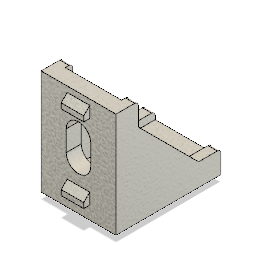
2020 Corner Bracket v1 (Autodesk Fusion 360 design; units mm, degrees)
Autodesk Fusion 360 part; units mm, degrees
sketch "Sketch1" plane through (0, 0, 0) normal (1, 0, 0) x (0, 0, -1)
  line L0 (0, 0) -> (0, 28)
  line L1 (0, 28) -> (5, 28)
  line L2 (6, 27) -> (6, 22)
  line L3 (6, 22) -> (22, 6)
  line L4 (22, 6) -> (27, 6)
  line L5 (28, 5) -> (28, 0)
  line L6 (28, 0) -> (0, 0)
  line L7 (4, 4) -> (28, 4)
  line L8 (4, 4) -> (4, 28)
  arc A0 (6, 27) -> (5, 28) centre (5, 27) ccw
  arc A1 (28, 5) -> (27, 6) centre (27, 5) ccw
  line L9 (0, 26.5) -> (-1.6, 24.9)
  line L10 (-1.6, 24.9) -> (-1.6, 23.5)
  line L11 (-1.6, 23.5) -> (0, 23.5)
  line L12 (0, 6.5) -> (-1.6, 4.9)
  line L13 (-1.6, 4.9) -> (-1.6, 3.5)
  line L14 (-1.6, 3.5) -> (0, 3.5)
  line L15 (3.5, 0) -> (3.5, -1.6)
  line L16 (3.5, -1.6) -> (4.9, -1.6)
  line L17 (4.9, -1.6) -> (6.5, 0)
  line L18 (23.5, 0) -> (23.5, -1.6)
  line L19 (23.5, -1.6) -> (24.9, -1.6)
  line L20 (24.9, -1.6) -> (26.5, 0)
  line L21 (-56.6063, 27.9695) -> (-36.6063, 27.9695)
  line L22 (-36.6063, 27.9695) -> (-36.6063, -0.0305)
  line L23 (-36.6063, -0.0305) -> (-56.6063, -0.0305)
  line L24 (-56.6063, -0.0305) -> (-56.6063, 27.9695)
  line L25 (-54.1063, 3.9695) -> (-39.1063, 3.9695)
  line L26 (-39.1063, 3.9695) -> (-39.1063, 27.9695)
  line L27 (-39.1063, 27.9695) -> (-54.1063, 27.9695)
  line L28 (-54.1063, 27.9695) -> (-54.1063, 3.9695)
  line L29 (-49.7743, 13.4695) -> (-49.7743, 16.9695)
  arc A2 (-43.2743, 16.9695) -> (-49.7743, 16.9695) centre (-46.5243, 16.9695) ccw
  line L30 (-43.2743, 16.9695) -> (-43.2743, 13.4695)
  arc A3 (-49.7743, 13.4695) -> (-43.2743, 13.4695) centre (-46.5243, 13.4695) ccw
  line L31 (-49.5243, -1.6305) -> (-43.5243, -1.6305)
  line L32 (-43.5243, -1.6305) -> (-43.5243, -0.0305)
  line L33 (-43.5243, -0.0305) -> (-49.5243, -0.0305)
  line L34 (-49.5243, -0.0305) -> (-49.5243, -1.6305)
  point P0 (6, 28)
  point P1 (28, 6)
  dimension "d1" = 28
  dimension "d2" = 28
  dimension "d3" = 6
  dimension "d4" = 6
  dimension "d5" = 45
  dimension "d6" = 22
  dimension "d7" = 4
  dimension "d8" = 4
  dimension "d9" = 1
  dimension "d11" = 45
  dimension "d12" = 1.6
  dimension "d14" = 3
  dimension "d16" = 3
  dimension "d17" = 20
  dimension "d18" = 20
  dimension "d19" = 3
  dimension "d20" = 3
  dimension "d21" = 45
  dimension "d22" = 3.5
  dimension "d23" = 1.6
  dimension "d26" = 20
  dimension "d27" = 2.5
  dimension "d28" = 15
  dimension "d29" = 6.5
  dimension "d30" = 3.5
  dimension "d31" = 13.5
  dimension "d32" = 4
  dimension "d33" = 28
  dimension "d34" = 6
  dimension "d35" = 0.25
  dimension "d36" = 1.6
  dimension "d41" = 3.5
  constraint coincident L0.start L6.end
  constraint vertical L0
  constraint perpendicular L0 L1
  constraint perpendicular L1 L2
  constraint perpendicular L2 L4
  constraint perpendicular L4 L5
  constraint perpendicular L0 L6
  constraint coincident L5 L7.end
  constraint perpendicular L5 L7
  constraint coincident L1 L8.end
  constraint perpendicular L1 L8
  constraint coincident P0 L1
  constraint coincident P0 L2
  constraint tangent L1 A0
  constraint tangent L2 A0
  constraint coincident P1 L4
  constraint coincident P1 L5
  constraint tangent L4 A1
  constraint tangent L5 A1
  constraint equal A0 A1
  constraint coincident L0 L9.start
  constraint parallel L0 L10
  constraint coincident L0 L11.end
  constraint perpendicular L0 L11
  constraint coincident L0 L12.start
  constraint parallel L0 L13
  constraint coincident L0 L14.end
  constraint perpendicular L0 L14
  constraint collinear L10 L13
  constraint coincident L6 L15.start
  constraint perpendicular L6 L15
  constraint perpendicular L15 L16
  constraint coincident L6 L17.end
  constraint coincident L6 L18.start
  constraint perpendicular L6 L18
  constraint perpendicular L18 L19
  constraint coincident L6 L20.end
  constraint parallel L17 L20
  constraint collinear L16 L19
  constraint parallel L9 L12
  constraint horizontal L21
  constraint vertical L22
  constraint horizontal L23
  constraint vertical L24
  constraint horizontal L25
  constraint vertical L26
  constraint horizontal L27
  constraint vertical L28
  constraint coincident L21 L26.end
  constraint vertical L29
  constraint tangent L29 A2
  constraint tangent A2 L30
  constraint parallel L29 L30
  constraint tangent L30 A3
  constraint tangent L29 A3
  constraint horizontal L31
  constraint vertical L32
  constraint horizontal L33
  constraint vertical L34
  constraint coincident L23 L32.end
  measures "d1" distance of L0.start L0.end
  measures "d2" distance of L0.start L5.end
  measures "d3" distance of L0.end P0
  measures "d4" distance of P1 L5.end
  measures "d5" angle of L3 L4
  measures "d6" distance of L2.end L6
  measures "d7" distance of L6 L7
  measures "d8" distance of L0 L8
  measures "d9" radius of A0
  measures "d11" angle of L0 L9
  measures "d12" distance of L0 L10
  measures "d14" distance of L9.start L11
  measures "d16" distance of L12.start L14
  measures "d17" distance of L11 L14
  measures "d18" distance of L15 L18
  measures "d19" distance of L15 L17.end
  measures "d20" distance of L18.start L20.end
  measures "d21" angle of L6 L17
  measures "d22" distance of L0 L15
  measures "d23" distance of L6 L16
  measures "d26" distance of L21.start L21.end
  measures "d27" distance of L24 L28
  measures "d28" distance of L25.start L25.end
  measures "d29" distance of L29 L30
  measures "d30" distance of A2.centre A3.centre
  measures "d31" distance of L23 A3.centre
  measures "d32" distance of L23 L25
  measures "d33" distance of L21.start L23.end
  measures "d34" distance of L31.start L31.end
  measures "d35" distance of L29 L34
  measures "d36" distance of L23 L31
  measures "d41" distance of L6 L14
extrude "Extrude1" add sketch "Sketch1" along normal mid plane 20 contours L0 L1 L5 L6 L7 L8 | L1 L2 L3 L4 L5 L7 L8 A0 A1
extrude "Extrude2" cut sketch "Sketch1" along normal mid plane 15 contours L1 L2 L3 L4 L5 L7 L8 A0 A1
extrude "Extrude3" add sketch "Sketch1" along normal mid plane 6 contours L0 L12 L13 L14 | L6 L15 L16 L17 | L0 L9 L10 L11 | L6 L18 L19 L20
sketch "Sketch2" plane through (0, 0, -4) normal (0, 0, -1) x (-1, 0, 0)
  line L0 (-7.5, 4) -> (7.5, 4)
  line L1 (7.5, 4) -> (7.5, 28)
  line L2 (7.5, 28) -> (-7.5, 28)
  line L3 (-7.5, 28) -> (-7.5, 4)
  line L4 (-3.25, 12.5) -> (-3.25, 18)
  arc A0 (3.25, 18) -> (-3.25, 18) centre (0, 18) ccw
  line L5 (3.25, 18) -> (3.25, 12.5)
  arc A1 (-3.25, 12.5) -> (3.25, 12.5) centre (0, 12.5) ccw
  line L6 (-10, 0) -> (10, 0)
  point P0 (0, 28)
  dimension "d42" = 6.5
  dimension "d43" = 5.5
  dimension "d44" = 12.5
  constraint vertical L4
  constraint tangent L4 A0
  constraint tangent A0 L5
  constraint parallel L4 L5
  constraint tangent L5 A1
  constraint tangent L4 A1
  constraint midpoint L2 P0
  constraint vertical A0.centre P0
  measures "d42" distance of L4 L5
  measures "d43" distance of A0.centre A1.centre
  measures "d44" distance of A1.centre L6
extrude "Extrude4" cut sketch "Sketch2" against normal through all contours L4 A0 L5 A1
sketch "Sketch3" plane through (0, 4, 0) normal (0, 1, 0) x (-1, 0, 0)
  line L0 (-7.5, -28) -> (7.5, -28)
  line L1 (7.5, -28) -> (7.5, -4)
  line L2 (7.5, -4) -> (-7.5, -4)
  line L3 (-7.5, -4) -> (-7.5, -28)
  line L4 (3.25, -12.5) -> (3.25, -18)
  arc A0 (-3.25, -18) -> (3.25, -18) centre (0, -18) ccw
  line L5 (-3.25, -18) -> (-3.25, -12.5)
  arc A1 (3.25, -12.5) -> (-3.25, -12.5) centre (0, -12.5) ccw
  line L6 (10, 0) -> (-10, 0)
  point P0 (0, -28)
  dimension "d46" = 6.5
  dimension "d47" = 12.5
  dimension "d48" = 5.5
  constraint vertical L4
  constraint tangent L4 A0
  constraint tangent A0 L5
  constraint parallel L4 L5
  constraint tangent L5 A1
  constraint tangent L4 A1
  constraint midpoint L0 P0
  constraint vertical A0.centre P0
  measures "d46" distance of L4 L5
  measures "d47" distance of A1.centre L6
  measures "d48" distance of A0.centre A1.centre
extrude "Extrude5" cut sketch "Sketch3" against normal through all contours L4 A0 L5 A1
equation "d16 = d14"
equation "d18 = d17"
equation "d19 = d14"
equation "d20 = d14"
equation "d21 = d11"
equation "d22 = d41"
equation "d23 = d12"
